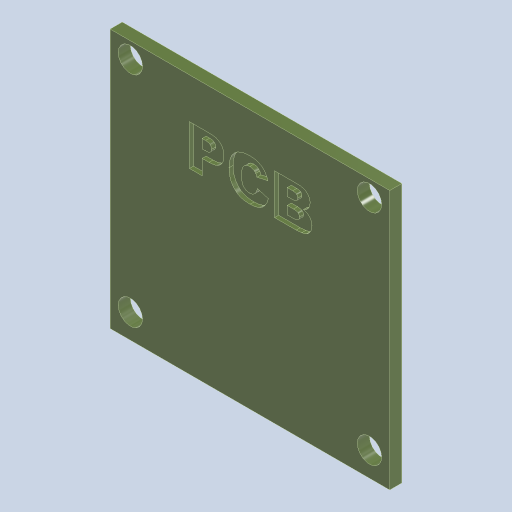
# Autodesk Inventor part: PCB_motor
Saved by Autodesk Inventor 2024.4 (Build 284460030, 460C)
## iProperties
Created: 2026-07-13
Part Number: PCB_motor
Material: Generic
Document SubType Name: Modeling
Designer: tooles01
Density: 1 g/cm^3
Appearance: Dark Olive
Author: tooles01
Autodesk Inventor part; units mm, degrees
ref_plane "YZ Plane" through (0, 0, 0) normal (1, 0, 0) x (0, 1, 0)
ref_plane "XZ Plane" through (0, 0, 0) normal (0, 1, 0) x (-1, 0, 0)
ref_plane "XY Plane" through (0, 0, 0) normal (0, 0, 1) x (1, 0, 0)
derived "door_front_01.ipt"
sketch "Sketch5: PCB footprint" plane through (0, 0, 0) normal (0, 0, 1) x (1, 0, 0)
  line L0 (-0.5, 81) -> (34, 81)
  line L1 (34, 81) -> (34, 49)
  line L2 (34, 49) -> (-0.5, 49)
  line L3 (-0.5, 49) -> (-0.5, 81)
  circle A0 centre (2, 79) radius 1.5
  circle A1 centre (31.5, 79) radius 1.5
  circle A2 centre (2, 52) radius 1.5
  circle A3 centre (31.5, 52) radius 1.5
  line L4 (2, 79) -> (31.5, 79) construction
  line L5 (31.5, 79) -> (31.5, 52) construction
  line L6 (31.5, 52) -> (2, 52) construction
  line L7 (2, 52) -> (2, 79) construction
  circle A4 centre (0, 30) radius 17.75
  line L8 (41, 0) -> (41, 85)
  point P0 (0, 0)
  point P1 (16.75, 79)
  point P2 (16.75, 81)
sketch "Sketch1: text" plane through (0, 0, 0) normal (0, 0, 1) x (1, 0, 0)
  line L0 (14.25, 76) -> (19.25, 76) construction
  line L1 (19.25, 76) -> (19.25, 71) construction
  line L2 (19.25, 71) -> (14.25, 71) construction
  line L3 (14.25, 71) -> (14.25, 76) construction
  line L4 (-0.5, 81) -> (34, 81) construction
  line L5 (9.2933, 76) -> (11.8631, 76)
  spline S0 degree 2 poles (11.8631, 76) (12.7004, 76) (13.5378, 75.2012) (13.5378, 74.4649) knots 0 0 0 1 2 2 2
  spline S1 degree 2 poles (13.5378, 74.4649) (13.5378, 73.7045) (12.6282, 72.8527) (11.6947, 72.8527) knots 0 0 0 1 2 2 2
  line L6 (11.6947, 72.8527) -> (10.8477, 72.8527)
  line L7 (10.8477, 72.8527) -> (10.8477, 71)
  line L8 (10.8477, 71) -> (9.2933, 71)
  line L9 (9.2933, 71) -> (9.2933, 76)
  line L10 (10.8477, 73.8681) -> (11.2231, 73.8681)
  spline S2 degree 2 poles (11.2231, 73.8681) (11.6706, 73.8681) (12.0315, 74.1809) (12.0315, 74.4216) knots 0 0 0 1 2 2 2
  spline S3 degree 2 poles (12.0315, 74.4216) (12.0315, 74.6574) (11.7187, 74.9846) (11.2856, 74.9846) knots 0 0 0 1 2 2 2
  line L11 (11.2856, 74.9846) -> (10.8477, 74.9846)
  line L12 (10.8477, 74.9846) -> (10.8477, 73.8681)
  line L13 (17.6764, 73.0452) -> (19.0286, 72.6362)
  spline S4 degree 2 poles (19.0286, 72.6362) (18.8939, 72.0683) (18.3068, 71.3032) (17.4358, 70.9134) (16.7668, 70.9134) knots 0 0 0 1 2 3 3 3
  spline S5 degree 2 poles (16.7668, 70.9134) (15.9487, 70.9134) (14.9189, 71.3898) (14.1682, 72.5833) (14.1682, 73.512) knots 0 0 0 1 2 3 3 3
  spline S6 degree 2 poles (14.1682, 73.512) (14.1682, 74.7536) (15.4868, 76.0866) (16.6947, 76.0866) knots 0 0 0 1 2 2 2
  spline S7 degree 2 poles (16.6947, 76.0866) (17.6379, 76.0866) (18.7158, 75.3215) (18.9805, 74.5322) knots 0 0 0 1 2 2 2
  line L14 (18.9805, 74.5322) -> (17.6138, 74.2291)
  spline S8 degree 2 poles (17.6138, 74.2291) (17.5416, 74.4552) (17.4646, 74.5611) knots 0 0 0 1 1 1
  spline S9 degree 2 poles (17.4646, 74.5611) (17.3347, 74.7392) (16.9593, 74.9317) (16.7283, 74.9317) knots 0 0 0 1 2 2 2
  spline S10 degree 2 poles (16.7283, 74.9317) (16.2086, 74.9317) (15.9295, 74.5082) knots 0 0 0 1 1 1
  spline S11 degree 2 poles (15.9295, 74.5082) (15.7178, 74.1954) (15.7178, 73.5217) knots 0 0 0 1 1 1
  spline S12 degree 2 poles (15.7178, 73.5217) (15.7178, 72.6891) (16.2231, 72.0731) (16.6802, 72.0731) knots 0 0 0 1 2 2 2
  spline S13 degree 2 poles (16.6802, 72.0731) (17.123, 72.0731) (17.5753, 72.5688) (17.6764, 73.0452) knots 0 0 0 1 2 2 2
  line L15 (19.789, 76) -> (22.6812, 76)
  spline S14 degree 2 poles (22.6812, 76) (23.403, 76) (24.1778, 75.283) (24.1778, 74.7536) knots 0 0 0 1 2 2 2
  spline S15 degree 2 poles (24.1778, 74.7536) (24.1778, 74.3109) (23.9035, 73.9933) knots 0 0 0 1 1 1
  spline S16 degree 2 poles (23.9035, 73.9933) (23.7158, 73.7815) (23.3597, 73.6564) knots 0 0 0 1 1 1
  spline S17 degree 2 poles (23.3597, 73.6564) (23.8987, 73.5265) (24.4088, 72.8961) (24.4088, 72.4196) knots 0 0 0 1 2 2 2
  spline S18 degree 2 poles (24.4088, 72.4196) (24.4088, 72.0346) (24.0479, 71.4139) (23.7351, 71.231) knots 0 0 0 1 2 2 2
  spline S19 degree 2 poles (23.7351, 71.231) (23.5378, 71.1203) (23.148, 71.0674) knots 0 0 0 1 1 1
  spline S20 degree 2 poles (23.148, 71.0674) (22.6234, 71) (22.455, 71) knots 0 0 0 1 1 1
  line L16 (22.455, 71) -> (19.789, 71)
  line L17 (19.789, 71) -> (19.789, 76)
  line L18 (21.3482, 72.0731) -> (22.1326, 72.0731)
  spline S21 degree 2 poles (22.1326, 72.0731) (22.532, 72.0731) (22.8592, 72.3571) (22.8592, 72.5929) knots 0 0 0 1 2 2 2
  spline S22 degree 2 poles (22.8592, 72.5929) (22.8592, 72.8142) (22.5368, 73.0837) (22.1326, 73.0837) knots 0 0 0 1 2 2 2
  line L19 (22.1326, 73.0837) -> (21.3482, 73.0837)
  line L20 (21.3482, 73.0837) -> (21.3482, 72.0731)
  line L21 (21.3482, 74.0366) -> (22.0171, 74.0366)
  spline S23 degree 2 poles (22.0171, 74.0366) (22.378, 74.0366) (22.6619, 74.2868) (22.6619, 74.5226) knots 0 0 0 1 2 2 2
  spline S24 degree 2 poles (22.6619, 74.5226) (22.6619, 74.7392) (22.378, 74.9846) (22.0267, 74.9846) knots 0 0 0 1 2 2 2
  line L22 (22.0267, 74.9846) -> (21.3482, 74.9846)
  line L23 (21.3482, 74.9846) -> (21.3482, 74.0366)
  point P0 (0, 0)
  point P1 (16.75, 76)
  point P2 (16.75, 81)
  dimension "d2" = 5
  dimension "d3" = 5
  constraints: 2 midpoint, 1 horizontal, 1 perpendicular, 1 vertical alignment, 2 other
  measures "d2" distance between parallel lines of L4 L0
  measures "d3" distance of L0.start L0.end
extrude "Ex1: base" add sketch "Sketch5: PCB footprint" against normal blind 1.5 contours L0 L1 L2 L3
extrude "Ex2: text" cut sketch "Sketch1: text" against normal blind 0.5
body "Solid1"
